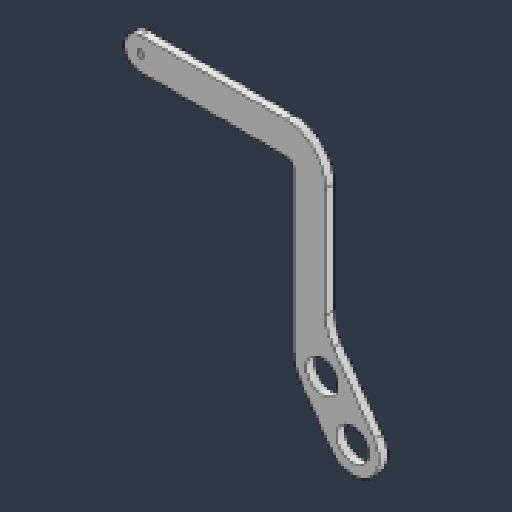
# Autodesk Inventor part: ARM,KICKER
Saved by Autodesk Inventor 2026 (Build 300175050, 175E)
## iProperties
Created: 2026-04-12
Part Number: ARM,KICKER
Material: Generic
Document SubType Name: Modeling
Designer: Jthib
Mass: 25.0533 g
Surface Area: 138.65 cm^2
Volume: 25.0533 cm^3
Density: 1 g/cm^3
Appearance: Default
Author: Jthib
Autodesk Inventor part; units mm, degrees
ref_plane "YZ Plane" through (0, 0, 0) normal (1, 0, 0) x (0, 1, 0)
ref_plane "XZ Plane" through (0, 0, 0) normal (0, 1, 0) x (-1, 0, 0)
ref_plane "XY Plane" through (0, 0, 0) normal (0, 0, 1) x (1, 0, 0)
sketch "Sketch1" plane through (0, 0, 0) normal (0, 0, 1) x (1, 0, 0)
  circle A0 centre (0, 0) radius 9.525
  line L0 (0, 9.525) -> (86.6775, 9.525)
  arc A1 (110.49, -14.2875) -> (86.6775, 9.525) centre (86.6775, -14.2875) ccw
  line L1 (110.49, -14.2875) -> (110.49, -90.0362)
  line L2 (110.49, -90.0362) -> (146.411, -125.9572)
  arc A2 (123.9604, -148.4079) -> (146.411, -125.9572) centre (135.1857, -137.1826) ccw
  line L3 (123.9604, -148.4079) -> (91.44, -115.8875)
  line L4 (91.44, -115.8875) -> (91.44, -14.2875)
  arc A3 (91.44, -14.2875) -> (86.6775, -9.525) centre (86.6775, -14.2875) ccw
  line L5 (86.6775, -9.525) -> (0, -9.525)
  circle A4 centre (135.1857, -137.1826) radius 9.525
  circle A5 centre (112.7351, -114.7319) radius 9.525
  line L6 (135.1857, -137.1826) -> (112.7351, -114.7319) construction
  dimension "d0" = 19.05
  dimension "d1" = 4.7625
  dimension "d4" = 91.44
  dimension "d5" = 101.6
  dimension "d6" = 31.75
  dimension "d7" = 50.8
  dimension "d8" = 19.05
  dimension "d9" = 19.05
  dimension "d10" = 31.75
  dimension "d11" = 135
  constraints: 14 end point, 8 point on circle, 8 tangent, 6 centre point, 3 parallel, 2 coincident, 2 perpendicular, 1 concentric, 1 horizontal
  measures "d0" diameter of A0
  measures "d1" radius of A3
  measures "d4" distance from line of L4 point (0, 0)
  measures "d5" distance of L3.end L4.end
  measures "d6" distance between parallel lines of L2 L3
  measures "d7" distance of L1.end L2.end
  measures "d8" diameter of A4
  measures "d9" diameter of A5
  measures "d10" distance of L6.start L6.end
  measures "d11" angle of L1 L2
extrude "Extrusion1" add sketch "Sketch1" along normal blind 4.7625
sketch "Sketch2" plane through (0, 0, 4.7625) normal (0, 0, 1) x (1, 0, 0)
  arc A0 (0, 9.525) -> (0, -9.525) centre (0, 0) ccw construction
  constraints: 1 coincident
hole "Hole1" at (0, 0, 4.7625) direction (0, 0, -1) diameter 3.9624 end through all thread size "10-32 UNF" class "2B" standard "ANSI Unified Screw Threads"
fillet "Fillet1" radius 25.4 2 edges at (110.49, -90.0362, 2.3813) (91.44, -115.8875, 2.3813)
body "Solid1"
